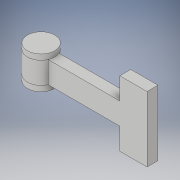
# Autodesk Inventor part: button_press_new
Saved by Autodesk Inventor 2017 (Build 210142000, 142)
## iProperties
Created: 2016-11-20
Part Number: button_press_new
Material: Generic
Document SubType Name: Modeling
Designer: radrajith
Density: 1 g/cm^3
Appearance: Default
Author: radrajith
Autodesk Inventor part; units mm, degrees
ref_plane "YZ Plane" through (0, 0, 0) normal (1, 0, 0) x (0, 1, 0)
ref_plane "XZ Plane" through (0, 0, 0) normal (0, 1, 0) x (-1, 0, 0)
ref_plane "XY Plane" through (0, 0, 0) normal (0, 0, 1) x (1, 0, 0)
sketch "Sketch1" plane through (0, 0, 0) normal (0, 1, 0) x (-1, 0, 0)
  line L0 (-22.9447, 5) -> (-22.9447, 0)
  line L1 (-22.9447, 0) -> (-8, 0)
  line L2 (-8, 0) -> (-8, 1.5)
  line L3 (-8, 1.5) -> (-4.7916, 1.5)
  line L4 (-8, 5) -> (-8, 3.5)
  line L5 (-8, 3.5) -> (-4.7916, 3.5)
  line L6 (-8, 5) -> (-22.9447, 5)
  arc A0 (-4.7916, 1.5) -> (-4.7916, 3.5) centre (-2.5, 2.5) ccw
  point P0 (0, 5)
  dimension "d1" = 5
  dimension "d2" = 1.5
  dimension "d3" = 1.5
  constraints: 14 end point, 2 point on circle, 1 centre point, 1 parallel, 1 perpendicular, 1 point on line
  measures "d1" distance of L0.end L0.start
  measures "d2" distance of L1.end L2.end
  measures "d3" distance of L4.end L4.start
extrude "Extrusion1" add sketch "Sketch1" along normal blind 4
sketch "Sketch6" plane through (8, 0, 0) normal (0, 0, -1) x (1, 0, 0)
  line L0 (0, 0) -> (0, -4) projected
  line L1 (0, -4) -> (14.9617, -4)
  line L2 (14.9617, -4) -> (14.9617, 1)
  line L3 (14.9617, 1) -> (0, 1)
  line L4 (0, 1) -> (0, -4)
  point P0 (-8, 0)
  constraints: 8 end point, 2 parallel, 1 horizontal, 1 perpendicular
extrude "Extrusion2" cut sketch "Sketch6" against normal blind 1.5
sketch "Sketch7" plane through (0, 4, 0) normal (0, 1, 0) x (-1, 0, 0)
  circle A0 centre (-2.5, 2.5) radius 2.5
  point P0 (0, 0)
  dimension "d8" = 5
  constraints: 1 centre point
  measures "d8" diameter of A0
extrude "Extrusion3" add sketch "Sketch7" along normal blind 1
sketch "Sketch8" plane through (0, 0, 0) normal (0, -1, 0) x (1, 0, 0)
  circle A0 centre (2.5, 2.5) radius 2.5
  point P0 (0, 0)
  dimension "d11" = 5
  constraints: 1 centre point
  measures "d11" diameter of A0
extrude "Extrusion4" add sketch "Sketch8" along normal blind 1
sketch "Sketch9" plane through (8, 0, 5) normal (0, 0, 1) x (1, 0, 0)
  line L0 (-3.2084, 0) -> (14.9447, 0) projected
  line L1 (-0.1278, 4) -> (14.9447, 4)
  line L2 (14.9447, 4) -> (14.9447, 0)
  line L3 (14.9447, 0) -> (-0.1278, 0)
  line L4 (-0.1278, 0) -> (-0.1278, 4)
  point P0 (-8, 0)
  constraints: 8 end point, 2 parallel, 1 horizontal, 1 perpendicular
extrude "Extrusion5" cut sketch "Sketch9" against normal blind 1.5
sketch "Sketch10" plane through (0, 4, 0) normal (0, 1, 0) x (1, 0, 0)
  line L0 (22.9447, -1.5) -> (22.9447, -3.5) projected
  line L1 (4.7916, -1.5) -> (22.9447, -1.5) projected
  line L2 (22.9447, -3.5) -> (17.9447, -3.5)
  line L3 (17.9447, -3.5) -> (17.9447, -1.5)
  line L4 (17.9447, -1.5) -> (22.9447, -1.5)
  line L5 (22.9447, -1.5) -> (22.9447, -3.5)
  point P0 (0, 0)
  dimension "d16" = 5
  constraints: 8 end point, 2 parallel, 1 horizontal, 1 perpendicular, 1 point on line
  measures "d16" distance of L3.end L4.end
extrude "Extrusion6" add sketch "Sketch10" along normal blind 4
sketch "Sketch11" plane through (0, 0, 0) normal (0, -1, 0) x (1, 0, 0)
  line L0 (22.9447, 1.5) -> (17.9447, 1.5) projected
  line L1 (17.9447, 3.5) -> (22.9447, 3.5) projected
  line L2 (22.9447, 1.5) -> (17.9447, 1.5)
  line L3 (17.9447, 1.5) -> (17.9447, 3.5)
  line L4 (17.9447, 3.5) -> (22.9447, 3.5)
  line L5 (22.9447, 3.5) -> (22.9447, 1.5)
  point P0 (0, 0)
  constraints: 8 end point, 2 parallel, 1 horizontal, 1 perpendicular
extrude "Extrusion7" add sketch "Sketch11" along normal blind 4
body "Solid1"
